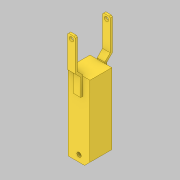
# Autodesk Inventor part: B5-A1
Saved by Autodesk Inventor 2018.1 (Build 221171000, 171)
## iProperties
Created: 2018-06-23
Part Number: B5-A1
Material: Všeobecné
Document SubType Name: Modeling
Designer: PS
Density: 1 g/cm^3
Appearance: Výchozí
Author: PS
Autodesk Inventor part; units mm, degrees
ref_plane "YZ Plane" through (0, 0, 0) normal (1, 0, 0) x (0, 1, 0)
ref_plane "XZ Plane" through (0, 0, 0) normal (0, 1, 0) x (-1, 0, 0)
ref_plane "XY Plane" through (0, 0, 0) normal (0, 0, 1) x (1, 0, 0)
sketch "Náčrt1" plane through (0, 0, 0) normal (0, 0, 1) x (1, 0, 0)
  line L0 (-100, -100) -> (100, -100)
  line L1 (100, -100) -> (100, 100)
  line L2 (100, 100) -> (-100, 100)
  line L3 (-100, 100) -> (-100, -100)
  line L4 (-100, -100) -> (100, 100) construction
  line L5 (100, -100) -> (-100, 100) construction
  point P0 (0, 0)
  dimension "d0" = 200
  constraints: 12 end point, 2 midpoint, 2 parallel, 2 perpendicular, 1 horizontal
  measures "d0" distance of L1.end L2.end
extrude "Vysunutí1" add sketch "Náčrt1" along normal blind 700
sketch "Náčrt2" plane through (0, 0, 0) normal (1, 0, 0) x (0, 1, 0)
  line L0 (-100, 0) -> (-100, 700) projected
  line L1 (-150, 760) -> (-150, 1045)
  line L2 (-120, 681.7157) -> (-120, 540)
  line L3 (-100, 700) -> (100, 700) projected
  line L4 (0, 700) -> (0, 773.8359) construction
  line L5 (-100, 0) -> (100, 0) projected
  line L6 (-100, 540) -> (-100, 710)
  line L7 (-100, 710) -> (-150, 760)
  line L8 (-170, 1045) -> (-170, 751.7157)
  line L9 (-170, 751.7157) -> (-120, 701.7157)
  line L10 (-120, 701.7157) -> (-120, 540)
  line L11 (-170, 1045) -> (-150, 1045)
  line L12 (-120, 540) -> (-100, 540)
  line L13 (-170, 1010) -> (-150, 1010) construction
  point P0 (0, 0)
  dimension "d5" = 150
  dimension "d22" = 135
  dimension "d24" = 20
  dimension "d26" = 10
  dimension "d35" = 345
  dimension "d36" = 35
  constraints: 22 end point, 4 point on line, 2 perpendicular, 1 horizontal, 1 midpoint, 1 vertical, 2 other
  measures "d5" distance between parallel lines of L1 L4
  measures "d22" angle of L1 L7
  measures "d24" distance between parallel lines of L1 L8
  measures "d26" distance from line of L3 L6.end
  measures "d35" distance between parallel lines of L3 L11
  measures "d36" distance between parallel lines of L13 L11
extrude "Vysunutí2" add sketch "Náčrt2" along normal mid plane 70
sketch "Náčrt3" plane through (-30, -170, 712.0978) normal (0, -1, 0) x (1, 0, 0)
  line L0 (-5, 332.9022) -> (65, 332.9022) projected
  line L1 (30, 332.9022) -> (30, 269.5637) construction
  circle A0 centre (30, 297.9022) radius 20
  point P0 (30, -712.0978)
  dimension "d11" = 40
  dimension "d12" = 35
  dimension "d25" = 70
  constraints: 2 end point, 1 centre point, 1 midpoint, 1 point on line, 1 vertical
  measures "d11" diameter of A0
  measures "d12" distance from line of A0.centre L0
  measures "d25" distance of L0.start L0.end
extrude "Vysunutí3" cut sketch "Náčrt3" against normal blind 60
chamfer "Zkosení1" distance 10 angle 45 2 edges at (35, -160, 1045) (-35, -160, 1045)
mirror "Zrcadlit1" about plane through (0, 0, 0) normal (0, 1, 0)
sketch "Náčrt4" plane through (-100, -100, 0) normal (0, -1, 0) x (1, 0, 0)
  circle A0 centre (100, 1010) radius 20 projected
  circle A1 centre (100, 60) radius 20
  line L0 (0, 0) -> (200, 0) projected
  line L1 (100, 0) -> (100, 549.2134) construction
  dimension "d27" = 40
  dimension "d28" = 60
  dimension "d29" = 950
  constraints: 2 end point, 1 centre point, 1 point on line, 1 vertical
  measures "d27" diameter of A1
  measures "d28" distance from line of A1.centre L0
  measures "d29" distance of A1.centre A0.centre
extrude "Vysunutí4" cut sketch "Náčrt4" against normal through all contours A1
chamfer "Zkosení2" distance 50 angle 45 1 edges at (100, 0, 0)
equation "\"d12\" = 0.5 * d25"
